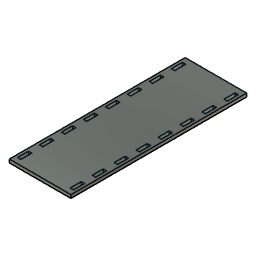
Slingshot Base (Autodesk Fusion 360 design; units mm, degrees)
Autodesk Fusion 360 part; units mm, degrees
note: some values were not read from the file. Set by a fixed rule: which sketch regions a step uses.
sketch "Sketch1" plane through (0, 0, 0) normal (0, 0, 1) x (1, 0, 0)
  line L0 (0, 0) -> (28, 0)
  line L1 (28, 0) -> (28, 160)
  line L2 (28, 160) -> (0, 160)
  line L3 (0, 160) -> (0, 0) construction
  line L4 (20, 0) -> (20, 160) construction
  line L5 (22.5, 155) -> (25.5, 155)
  line L6 (25.5, 155) -> (25.5, 145)
  line L7 (25.5, 145) -> (22.5, 145)
  line L8 (22.5, 145) -> (22.5, 155)
  line L9 (25.5, 155) -> (25.5, 160) construction
  line L10 (25.5, 155) -> (28, 155) construction
  line L11 (22.5, 135) -> (25.5, 135)
  line L12 (25.5, 135) -> (25.5, 125)
  line L13 (25.5, 125) -> (22.5, 125)
  line L14 (22.5, 125) -> (22.5, 135)
  line L15 (24, 145) -> (24, 135) construction
  line L16 (22.5, 105) -> (22.5, 115)
  line L17 (25.5, 105) -> (22.5, 105)
  line L18 (25.5, 115) -> (25.5, 105)
  line L19 (22.5, 115) -> (25.5, 115)
  line L20 (24, 115) -> (24, 125) construction
  line L21 (25.5, 95) -> (25.5, 85)
  line L22 (25.5, 85) -> (22.5, 85)
  line L23 (22.5, 85) -> (22.5, 95)
  line L24 (22.5, 95) -> (25.5, 95)
  line L25 (24, 95) -> (24, 105) construction
  line L26 (25.5, 95) -> (28, 95) construction
  line L27 (22.5, 75) -> (25.5, 75)
  line L28 (25.5, 75) -> (25.5, 65)
  line L29 (25.5, 65) -> (22.5, 65)
  line L30 (22.5, 65) -> (22.5, 75)
  line L31 (22.5, 55) -> (25.5, 55)
  line L32 (25.5, 55) -> (25.5, 45)
  line L33 (25.5, 45) -> (22.5, 45)
  line L34 (22.5, 45) -> (22.5, 55)
  line L35 (24, 85) -> (24, 75) construction
  line L36 (25.5, 75) -> (28, 75) construction
  line L37 (25.5, 55) -> (28, 55) construction
  line L38 (24, 55) -> (24, 65) construction
  line L39 (25.5, 135) -> (28, 135) construction
  line L40 (25.5, 115) -> (28, 115) construction
  line L41 (22.5, 35) -> (25.5, 35)
  line L42 (25.5, 35) -> (25.5, 25)
  line L43 (25.5, 25) -> (22.5, 25)
  line L44 (22.5, 25) -> (22.5, 35)
  line L45 (25.5, 35) -> (28, 35) construction
  line L46 (24, 45) -> (24, 35) construction
  line L47 (22.5, 15) -> (25.5, 15)
  line L48 (25.5, 15) -> (25.5, 5)
  line L49 (25.5, 5) -> (22.5, 5)
  line L50 (22.5, 5) -> (22.5, 15)
  line L51 (24, 15) -> (24, 25) construction
  line L52 (25.5, 15) -> (28, 15) construction
  line L53 (-25.5, 75) -> (-28, 75) construction
  line L54 (-25.5, 75) -> (-25.5, 65)
  line L55 (-20, 0) -> (-20, 160) construction
  line L56 (-24, 85) -> (-24, 75) construction
  line L57 (-25.5, 115) -> (-28, 115) construction
  line L58 (-22.5, 45) -> (-22.5, 55)
  line L59 (-25.5, 145) -> (-22.5, 145)
  line L60 (-25.5, 135) -> (-28, 135) construction
  line L61 (-22.5, 115) -> (-25.5, 115)
  line L62 (-25.5, 105) -> (-22.5, 105)
  line L63 (-22.5, 65) -> (-22.5, 75)
  line L64 (0, 160) -> (0, 0) construction
  line L65 (-24, 45) -> (-24, 35) construction
  line L66 (-25.5, 135) -> (-25.5, 125)
  line L67 (-28, 160) -> (0, 160)
  line L68 (-25.5, 155) -> (-28, 155) construction
  line L69 (-25.5, 125) -> (-22.5, 125)
  line L70 (-25.5, 55) -> (-28, 55) construction
  line L71 (-24, 15) -> (-24, 25) construction
  line L72 (-22.5, 135) -> (-25.5, 135)
  line L73 (-25.5, 15) -> (-28, 15) construction
  line L74 (-22.5, 75) -> (-25.5, 75)
  line L75 (-25.5, 115) -> (-25.5, 105)
  line L76 (-25.5, 155) -> (-25.5, 145)
  line L77 (-22.5, 105) -> (-22.5, 115)
  line L78 (-24, 115) -> (-24, 125) construction
  line L79 (-25.5, 95) -> (-25.5, 85)
  line L80 (-25.5, 55) -> (-25.5, 45)
  line L81 (-28, 0) -> (-28, 160)
  line L82 (-22.5, 155) -> (-25.5, 155)
  line L83 (-22.5, 85) -> (-22.5, 95)
  line L84 (-24, 95) -> (-24, 105) construction
  line L85 (-25.5, 15) -> (-25.5, 5)
  line L86 (-25.5, 5) -> (-22.5, 5)
  line L87 (-25.5, 155) -> (-25.5, 160) construction
  line L88 (-25.5, 35) -> (-28, 35) construction
  line L89 (-22.5, 25) -> (-22.5, 35)
  line L90 (-22.5, 35) -> (-25.5, 35)
  line L91 (-25.5, 95) -> (-28, 95) construction
  line L92 (-25.5, 25) -> (-22.5, 25)
  line L93 (-22.5, 95) -> (-25.5, 95)
  line L94 (-25.5, 45) -> (-22.5, 45)
  line L95 (-22.5, 125) -> (-22.5, 135)
  line L96 (-22.5, 145) -> (-22.5, 155)
  line L97 (-24, 145) -> (-24, 135) construction
  line L98 (-22.5, 55) -> (-25.5, 55)
  line L99 (-25.5, 65) -> (-22.5, 65)
  line L100 (-25.5, 85) -> (-22.5, 85)
  line L101 (-24, 55) -> (-24, 65) construction
  line L102 (-25.5, 35) -> (-25.5, 25)
  line L103 (0, 0) -> (-28, 0)
  line L104 (-22.5, 15) -> (-25.5, 15)
  line L105 (-22.5, 5) -> (-22.5, 15)
  point P0 (24, 115)
  point P1 (24, 95)
  point P2 (24, 95)
  point P3 (-24, 115)
  point P4 (-24, 95)
  point P5 (-24, 95)
  dimension "d3" = 160
  dimension "d4" = 28
  dimension "d5" = 5
  dimension "d6" = 2.5
  dimension "d7" = 10
  dimension "d8" = 3
  dimension "d9" = 10
  constraint coincident L0.start L3.end
  constraint horizontal L0
  constraint perpendicular L0 L1
  constraint perpendicular L1 L2
  constraint perpendicular L0 L3
  constraint coincident L0 L4.start
  constraint coincident L2 L4.end
  constraint perpendicular L2 L4
  constraint horizontal L5
  constraint vertical L6
  constraint horizontal L7
  constraint vertical L8
  constraint coincident L2 L9.end
  constraint perpendicular L2 L9
  constraint coincident L1 L10.end
  constraint perpendicular L1 L10
  constraint horizontal L11
  constraint vertical L12
  constraint horizontal L13
  constraint vertical L14
  constraint midpoint L7 L15.start
  constraint midpoint L11 L15.end
  constraint perpendicular L11 L15
  constraint equal L8 L14
  constraint equal L7 L13
  constraint horizontal L19
  constraint vertical L18
  constraint horizontal L17
  constraint vertical L16
  constraint midpoint P0 L19
  constraint coincident P0 L20.start
  constraint midpoint L13 L20.end
  constraint perpendicular L13 L20
  constraint equal L15 L20
  constraint equal L14 L16
  constraint equal L13 L17
  constraint horizontal L24
  constraint vertical L21
  constraint horizontal L22
  constraint vertical L23
  constraint midpoint P2 L24
  constraint coincident P2 P1
  constraint midpoint L17 L25.end
  constraint equal L20 L25
  constraint equal L16 L23
  constraint equal L17 L22
  constraint coincident L1 L26.end
  constraint perpendicular L1 L26
  constraint equal L10 L26
  constraint horizontal L27
  constraint vertical L28
  constraint horizontal L29
  constraint vertical L30
  constraint horizontal L31
  constraint vertical L32
  constraint horizontal L33
  constraint vertical L34
  constraint midpoint L22 L35.start
  constraint midpoint L27 L35.end
  constraint coincident L1 L36.end
  constraint perpendicular L1 L36
  constraint equal L26 L36
  constraint equal L22 L27
  constraint equal L23 L30
  constraint equal L25 L35
  constraint coincident L1 L37.end
  constraint perpendicular L1 L37
  constraint midpoint L31 L38.start
  constraint midpoint L29 L38.end
  constraint equal L36 L37
  constraint equal L29 L31
  constraint equal L35 L38
  constraint equal L30 L34
  constraint coincident L1 L39.end
  constraint perpendicular L1 L39
  constraint coincident L1 L40.end
  constraint perpendicular L1 L40
  constraint horizontal L41
  constraint vertical L42
  constraint horizontal L43
  constraint vertical L44
  constraint coincident L1 L45.end
  constraint perpendicular L1 L45
  constraint midpoint L33 L46.start
  constraint midpoint L41 L46.end
  constraint equal L37 L45
  constraint equal L38 L46
  constraint equal L33 L41
  constraint equal L34 L44
  constraint horizontal L47
  constraint vertical L48
  constraint horizontal L49
  constraint vertical L50
  constraint midpoint L47 L51.start
  constraint midpoint L43 L51.end
  constraint coincident L1 L52.end
  constraint perpendicular L1 L52
  constraint equal L45 L52
  constraint equal L43 L47
  constraint equal L44 L50
  constraint equal L46 L51
  constraint symmetric L0.start L3 L64.end
  constraint symmetric L0.end L3 L81.start
  constraint symmetric L1.end L3 L67.start
  constraint symmetric L2.end L3 L64.start
  constraint symmetric L3 L4.start L55.start
  constraint symmetric L3 L4.end L55.end
  constraint symmetric L3 L5.start L82.start
  constraint symmetric L3 L5.end L68.start
  constraint symmetric L3 L6.end L59.start
  constraint symmetric L3 L7.end L59.end
  constraint symmetric L3 L9.end L87.end
  constraint symmetric L3 L10.end L68.end
  constraint symmetric L3 L11.start L72.start
  constraint symmetric L3 L11.end L60.start
  constraint symmetric L3 L12.end L66.end
  constraint symmetric L3 L13.end L69.end
  constraint symmetric L3 L15.start L97.start
  constraint symmetric L3 L15.end L97.end
  constraint symmetric L3 L16.start L62.end
  constraint symmetric L3 P0 P3
  constraint symmetric L3 L18.start L57.start
  constraint symmetric L3 L17.start L62.start
  constraint symmetric L3 L16.end L61.start
  constraint symmetric L3 L20.end L78.end
  constraint symmetric L3 P2 P5
  constraint symmetric L3 L22.end L83.start
  constraint symmetric L3 L21.end L79.end
  constraint symmetric L3 L23.end L83.end
  constraint symmetric L3 L21.start L79.start
  constraint symmetric L3 L25.end L84.end
  constraint symmetric L3 L26.end L91.end
  constraint symmetric L3 L27.start L63.end
  constraint symmetric L3 L27.end L53.start
  constraint symmetric L3 L28.end L54.end
  constraint symmetric L3 L29.end L63.start
  constraint symmetric L3 L31.start L58.end
  constraint symmetric L3 L31.end L70.start
  constraint symmetric L3 L32.end L80.end
  constraint symmetric L3 L33.end L58.start
  constraint symmetric L3 L35.start L56.start
  constraint symmetric L3 L35.end L56.end
  constraint symmetric L3 L36.end L53.end
  constraint symmetric L3 L37.end L70.end
  constraint symmetric L3 L38.start L101.start
  constraint symmetric L3 L38.end L101.end
  constraint symmetric L3 L39.end L60.end
  constraint symmetric L3 L40.end L57.end
  constraint symmetric L3 L41.start L89.end
  constraint symmetric L3 L41.end L88.start
  constraint symmetric L3 L42.end L92.start
  constraint symmetric L3 L43.end L89.start
  constraint symmetric L3 L45.end L88.end
  constraint symmetric L3 L46.start L65.start
  constraint symmetric L3 L46.end L65.end
  constraint symmetric L3 L47.start L104.start
  constraint symmetric L3 L47.end L73.start
  constraint symmetric L3 L48.end L85.end
  constraint symmetric L3 L49.end L86.end
  constraint symmetric L3 L51.start L71.start
  constraint symmetric L3 L51.end L71.end
  constraint symmetric L3 L52.end L73.end
  measures "d3" distance of L0.end L1.end
  measures "d4" distance of L1.end L2.end
  measures "d5" distance of L5.end L9.end
  measures "d6" distance of L5.end L10.end
  measures "d7" distance of L5.start L7.end
  measures "d8" distance of L6.end L7.end
  measures "d9" distance of L15.start L15.end
extrude "Extrude1" add sketch "Sketch1" along normal blind 3
sketch "Sketch2" plane through (0, 0, 3) normal (0, 0, 1) x (-1, 0, 0)
  line L0 (-22.5, -105) -> (-22.5, -115)
  line L1 (-22.5, -115) -> (-25.5, -115)
  line L2 (-25.5, -115) -> (-25.5, -105)
  line L3 (-25.5, -105) -> (-22.5, -105)
  line L4 (-22.5, -85) -> (-22.5, -95)
  line L5 (-22.5, -95) -> (-25.5, -95)
  line L6 (-25.5, -95) -> (-25.5, -85)
  line L7 (-25.5, -85) -> (-22.5, -85)
  line L8 (-25.5, -145) -> (-22.5, -145)
  line L9 (-22.5, -145) -> (-22.5, -155)
  line L10 (-22.5, -155) -> (-25.5, -155)
  line L11 (-25.5, -155) -> (-25.5, -145)
  line L12 (-25.5, -65) -> (-22.5, -65)
  line L13 (-22.5, -65) -> (-22.5, -75)
  line L14 (-22.5, -75) -> (-25.5, -75)
  line L15 (-25.5, -75) -> (-25.5, -65)
  line L16 (-25.5, -125) -> (-22.5, -125)
  line L17 (-22.5, -125) -> (-22.5, -135)
  line L18 (-22.5, -135) -> (-25.5, -135)
  line L19 (-25.5, -135) -> (-25.5, -125)
  line L20 (-25.5, -25) -> (-22.5, -25)
  line L21 (-22.5, -25) -> (-22.5, -35)
  line L22 (-22.5, -35) -> (-25.5, -35)
  line L23 (-25.5, -35) -> (-25.5, -25)
  line L24 (-25.5, -5) -> (-22.5, -5)
  line L25 (-22.5, -5) -> (-22.5, -15)
  line L26 (-22.5, -15) -> (-25.5, -15)
  line L27 (-25.5, -15) -> (-25.5, -5)
  line L28 (22.5, -115) -> (22.5, -105)
  line L29 (22.5, -105) -> (25.5, -105)
  line L30 (25.5, -105) -> (25.5, -115)
  line L31 (25.5, -115) -> (22.5, -115)
  line L32 (22.5, -15) -> (22.5, -5)
  line L33 (22.5, -5) -> (25.5, -5)
  line L34 (25.5, -5) -> (25.5, -15)
  line L35 (25.5, -15) -> (22.5, -15)
  line L36 (25.5, -25) -> (25.5, -35)
  line L37 (25.5, -35) -> (22.5, -35)
  line L38 (22.5, -35) -> (22.5, -25)
  line L39 (22.5, -25) -> (25.5, -25)
  line L40 (22.5, -85) -> (25.5, -85)
  line L41 (25.5, -85) -> (25.5, -95)
  line L42 (25.5, -95) -> (22.5, -95)
  line L43 (22.5, -95) -> (22.5, -85)
  line L44 (22.5, -65) -> (25.5, -65)
  line L45 (25.5, -65) -> (25.5, -75)
  line L46 (25.5, -75) -> (22.5, -75)
  line L47 (22.5, -75) -> (22.5, -65)
  line L48 (25.5, -55) -> (22.5, -55)
  line L49 (22.5, -55) -> (22.5, -45)
  line L50 (22.5, -45) -> (25.5, -45)
  line L51 (25.5, -45) -> (25.5, -55)
  line L52 (22.5, -155) -> (22.5, -145)
  line L53 (22.5, -145) -> (25.5, -145)
  line L54 (25.5, -145) -> (25.5, -155)
  line L55 (25.5, -155) -> (22.5, -155)
  line L56 (22.5, -135) -> (22.5, -125)
  line L57 (22.5, -125) -> (25.5, -125)
  line L58 (25.5, -125) -> (25.5, -135)
  line L59 (25.5, -135) -> (22.5, -135)
  line L60 (-25.5, -45) -> (-22.5, -45)
  line L61 (-22.5, -45) -> (-22.5, -55)
  line L62 (-22.5, -55) -> (-25.5, -55)
  line L63 (-25.5, -55) -> (-25.5, -45)
  line L64 (-28, 0) -> (-28, -160)
  line L65 (-28, -160) -> (28, -160)
  line L66 (28, -160) -> (28, 0)
  line L67 (28, 0) -> (-28, 0)
